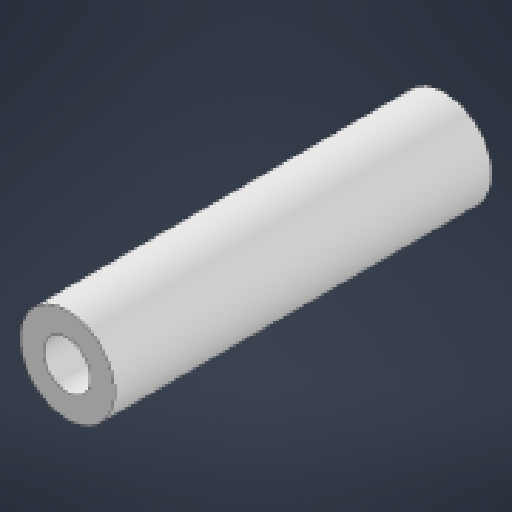
# Autodesk Inventor part: spacer_etage
Saved by Autodesk Inventor 2024 (Build 280153000, 153)
## iProperties
Created: 2026-03-25
Part Number: spacer_etage
Material: Generic
Document SubType Name: Modeling
Designer: schar
Density: 1 g/cm^3
Appearance: Default
Author: schar
Autodesk Inventor part; units mm, degrees
ref_plane "YZ Plane" through (0, 0, 0) normal (1, 0, 0) x (0, 1, 0)
ref_plane "XZ Plane" through (0, 0, 0) normal (0, 1, 0) x (-1, 0, 0)
ref_plane "XY Plane" through (0, 0, 0) normal (0, 0, 1) x (1, 0, 0)
sketch "Sketch1" plane through (0, 0, 0) normal (0, 0, 1) x (1, 0, 0)
  arc A0 (-98.923, 4.3301) -> (-98.923, -4.3301) centre (-96.423, 0) ccw projected
  arc A1 (93.923, -115.6699) -> (101.423, -111.3397) centre (96.423, -111.3397) ccw projected
  arc A2 (101.423, 111.3397) -> (93.923, 115.6699) centre (96.423, 111.3397) ccw projected
  line L0 (-96.423, 0) -> (-76.423, 0)
  circle A3 centre (-76.423, 0) radius 2.5
  circle A4 centre (-76.423, 0) radius 5
  line L1 (-82.9845, -199.4033) -> (136.5211, 180.7915)
  line L2 (-82.9845, 199.4033) -> (136.5211, -180.7915)
  point P0 (0, 0)
  point P1 (32.141, 0)
  dimension "d0" = 20
  dimension "d1" = 5
  dimension "d2" = 10
  constraints: 6 end point, 2 centre point, 2 coincident, 2 point on line, 1 horizontal, 6 other
  measures "d0" distance of L0.start L0.end
  measures "d1" diameter of A3
  measures "d2" diameter of A4
extrude "Extrusion1" add sketch "Sketch1" along normal blind 40
body "Solid1"
